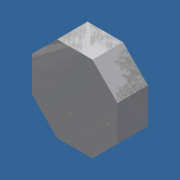
# Autodesk Inventor part: Oktagon
Saved by Autodesk Inventor 2018.2 (Build 222227000, 227)
## iProperties
Created: 2018-10-01
Part Number: Oktagon
Material: Kst - PVC (rigid/white)
Document SubType Name: Modeling
Designer: N.Grubert
Density: 1.38 g/cm^3
Appearance: Glatt - weiß
Fläche: 0 cm²
Gewicht: 0 g
Material: geeigneten Werkstoff auswählen !
Dateiname: P:\INVENTOR\Inventor 2018\Templates\ILT\Norm.ipt
Bez_eng: bolt
Bez_french: boulon
Author: N.Grubert
Autodesk Inventor part; units mm, degrees
ref_plane "YZ Plane" through (0, 0, 0) normal (1, 0, 0) x (0, 1, 0)
ref_plane "XZ Plane" through (0, 0, 0) normal (0, 1, 0) x (-1, 0, 0)
ref_plane "XY Plane" through (0, 0, 0) normal (0, 0, 1) x (1, 0, 0)
sketch "Skizze4" plane through (0, 0, 0) normal (0, 1, 0) x (-1, 0, 0)
  line L0 (98, 0) -> (-98, 0) construction
  line L1 (0, -98) -> (0, 98) construction
  line L2 (27, 37.5) -> (-27, 37.5) construction
  line L3 (-27, 37.5) -> (-27, -37.5) construction
  line L4 (-27, -37.5) -> (27, -37.5) construction
  line L5 (27, -37.5) -> (27, 37.5) construction
  line L6 (70, -28.9949) -> (28.9949, -70)
  line L7 (28.9949, -70) -> (-28.9949, -70)
  line L8 (-28.9949, -70) -> (-70, -28.9949)
  line L9 (-70, -28.9949) -> (-70, 28.9949)
  line L10 (-70, 28.9949) -> (-28.9949, 70)
  line L11 (-28.9949, 70) -> (28.9949, 70)
  line L12 (28.9949, 70) -> (70, 28.9949)
  line L13 (70, 28.9949) -> (70, -28.9949)
  line L14 (67.5, -27.9594) -> (27.9594, -67.5)
  line L15 (27.9594, -67.5) -> (-27.9594, -67.5)
  line L16 (-27.9594, -67.5) -> (-67.5, -27.9594)
  line L17 (-67.5, -27.9594) -> (-67.5, 27.9594)
  line L18 (-67.5, 27.9594) -> (-27.9594, 67.5)
  line L19 (-27.9594, 67.5) -> (27.9594, 67.5)
  line L20 (27.9594, 67.5) -> (67.5, 27.9594)
  line L21 (67.5, 27.9594) -> (67.5, -27.9594)
  point P0 (0, 0)
  point P1 (0, 0)
  dimension "d4" = 75
  dimension "d5" = 54
  dimension "d7" = 2.5
  dimension "d12" = 135
  constraints: 40 end point, 2 parallel, 1 coincident, 1 horizontal, 1 perpendicular, 27 other
  measures "d4" distance between parallel lines of L4 L2
  measures "d5" distance between parallel lines of L3 L5
  measures "d7" distance between parallel lines of L13 L21
  measures "d12" distance between parallel lines of L17 L21
extrude "Extrusion2" add sketch "Skizze4" along normal blind 45
sketch "Skizze5" plane through (0, 0, 0) normal (0, -1, 0) x (1, 0, 0)
  line L0 (27.9594, -67.5) -> (-27.9594, -67.5) projected
  line L1 (-27.9594, -67.5) -> (-67.5, -27.9594) projected
  line L2 (-67.5, -27.9594) -> (-67.5, 27.9594) projected
  line L3 (-67.5, 27.9594) -> (-27.9594, 67.5) projected
  line L4 (-27.9594, 67.5) -> (27.9594, 67.5) projected
  line L5 (27.9594, 67.5) -> (67.5, 27.9594) projected
  line L6 (67.5, 27.9594) -> (67.5, -27.9594) projected
  line L7 (67.5, -27.9594) -> (27.9594, -67.5) projected
  line L8 (-70, -28.9949) -> (-28.9949, -70) projected
  line L9 (-28.9949, -70) -> (28.9949, -70) projected
  line L10 (28.9949, -70) -> (70, -28.9949) projected
  line L11 (70, -28.9949) -> (70, 28.9949) projected
  line L12 (70, 28.9949) -> (28.9949, 70) projected
  line L13 (28.9949, 70) -> (-28.9949, 70) projected
  line L14 (-28.9949, 70) -> (-70, 28.9949) projected
  line L15 (-70, 28.9949) -> (-70, -28.9949) projected
  point P0 (0, 0)
extrude "Extrusion3" add sketch "Skizze5" along normal blind 5 contours L0 L1 L2 L3 L4 L5 L6 L7 | L15 L14 L13 L12 L11 L10 L9 L8
